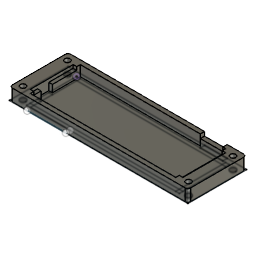
case-bottom (Autodesk Fusion 360 design; units mm, degrees)
part number: 2025-11-21-15-01-15-450
part number: 2025-11-21-15-01-59-170
Autodesk Fusion 360 part; units mm, degrees
sketch "Sketch1" plane through (0, 0, 0) normal (0, 0, 1) x (1, 0, 0) in component "guilty pad case"
  line L0 (0, 0) -> (94.784, 0)
  line L1 (94.784, 0) -> (94.784, -31)
  line L2 (94.784, -31) -> (0, -31)
  line L3 (0, -31) -> (0, 0)
  line L4 (-8, 2.7) -> (102.784, 2.7)
  line L5 (102.784, 2.7) -> (102.784, -33.7)
  line L6 (102.784, -33.7) -> (-8, -33.7)
  line L7 (-8, -33.7) -> (-8, 2.7)
  circle A0 centre (-4, -29.3) radius 1.7
  circle A1 centre (98.784, -29.3) radius 1.7
  circle A2 centre (98.784, -1.7) radius 1.7
  circle A3 centre (-4, -1.7) radius 1.7
  line L8 (3, -31) -> (27, -31)
  line L9 (27, -33.7) -> (3, -33.7)
  line L10 (90.784, 0) -> (76.784, 0)
  line L11 (76.784, 0) -> (76.784, 2.7)
  line L12 (76.784, 2.7) -> (90.784, 2.7)
  line L13 (90.784, 2.7) -> (90.784, 0)
  line L14 (92.534, 0) -> (92.534, -31)
  line L15 (2.25, 0) -> (2.25, -31)
  line L16 (0, -2.2) -> (94.784, -2.2)
  line L17 (0, -28.8) -> (94.784, -28.8)
  line L18 (0, -24.3) -> (2.25, -24.3)
  line L19 (0, -17.3) -> (2.25, -17.3)
  dimension "d4" = 36.4
  dimension "d5" = 110.784
  dimension "d6" = 94.784
  dimension "d7" = 31
  dimension "d9" = 3.4
  dimension "d10" = 4.4
  dimension "d11" = 4
  dimension "d12" = 3.4
  dimension "d13" = 4
  dimension "d14" = 4.4
  dimension "d15" = 3.4
  dimension "d16" = 4.4
  dimension "d17" = 4
  dimension "d18" = 3.4
  dimension "d19" = 4.4
  dimension "d20" = 4
  dimension "d21" = 2.7
  dimension "d22" = 8
  dimension "d23" = 24
  dimension "d24" = 2.7
  dimension "d26" = 4
  dimension "d27" = 14
  dimension "d32" = 2.25
  dimension "d33" = 2.25
  dimension "d73" = 2.2
  dimension "d74" = 2.2
  dimension "d77" = 4.5
  dimension "d78" = 7
  constraint horizontal L0
  constraint vertical L1
  constraint horizontal L2
  constraint vertical L3
  constraint coincident L0.start L3.end
  constraint horizontal L4
  constraint vertical L5
  constraint horizontal L6
  constraint vertical L7
  constraint horizontal L8
  constraint horizontal L9
  constraint coincident L2 L8.start
  constraint horizontal L10
  constraint vertical L11
  constraint horizontal L12
  constraint vertical L13
  constraint coincident L4 L11.end
  constraint coincident L0 L10.start
  constraint coincident L0 L14.start
  constraint coincident L2 L14.end
  constraint perpendicular L2 L14
  constraint coincident L0 L15.start
  constraint coincident L2 L15.end
  constraint perpendicular L2 L15
  constraint coincident L3 L16.start
  constraint coincident L1 L16.end
  constraint perpendicular L1 L16
  constraint coincident L3 L17.start
  constraint coincident L1 L17.end
  constraint perpendicular L1 L17
  constraint coincident L3 L18.start
  constraint coincident L15 L18.end
  constraint perpendicular L15 L18
  constraint coincident L3 L19.start
  constraint coincident L15 L19.end
  constraint perpendicular L15 L19
  measures "d4" distance of L4.start L6.end
  measures "d5" distance of L4.start L4.end
  measures "d6" distance of L0.start L0.end
  measures "d7" distance of L0.start L2.end
  measures "d9" diameter of A0
  measures "d10" distance of L6 A0.centre
  measures "d11" distance of L7 A0.centre
  measures "d12" diameter of A1
  measures "d13" distance of L5 A1.centre
  measures "d14" distance of L6 A1.centre
  measures "d15" diameter of A2
  measures "d16" distance of L4 A2.centre
  measures "d17" distance of L5 A2.centre
  measures "d18" diameter of A3
  measures "d19" distance of L4 A3.centre
  measures "d20" distance of L7 A3.centre
  measures "d21" distance of L2 L6
  measures "d22" distance of L1 L5
  measures "d23" distance of L8.start L8.end
  measures "d24" distance of L8.end L9.start
  measures "d26" distance of L0.end L13
  measures "d27" distance of L11 L13
  measures "d32" distance of L1 L14
  measures "d33" distance of L3 L15
  measures "d73" distance of L0 L16
  measures "d74" distance of L2 L17
  measures "d77" distance of L17 L18
  measures "d78" distance of L18 L19
extrude "Extrude2" add sketch "Sketch1" along normal blind 7.5 contours L0 L1 L2 L3 L4 L5 L6 L7 L8 L9 L11 L13 | L0 L3 L15 L16 | L0 L1 L14 L16 | L1 L2 L14 L17 | L2 L3 L15 L17 makes body 1 in component "guilty pad case"
extrude "Extrude3" add sketch "Sketch1" along normal blind 5.5 separate body contours L0 L3 L15 L16 | L3 L15 L16 L19 | L1 L14 L16 L17 | L0 L1 L14 L16 | L3 L15 L17 L18 | L1 L2 L14 L17 | L2 L3 L15 L17 makes body 2 at (0, -11.5333, 1.8333) makes body 3 at (94.784, -10.3333, 1.8333) makes body 4 at (0, -28.7667, 1.8333) in component "guilty pad case"
extrude "Extrude9" add sketch "Sketch1" along normal blind 1 contours L0 L1 L2 L3 L4 L5 L6 L7 L8 L9 L11 L13 | L0 L3 L15 L16 | L0 L10 L14 L15 L16 | L3 L15 L16 L19 | L0 L4 L10 L11 L12 L13 | L14 L15 L16 L17 | L3 L15 L18 L19 | L1 L14 L16 L17 | L0 L1 L14 L16 | L3 L15 L17 L18 | L1 L2 L14 L17 | L2 L8 L14 L15 L17 | L2 L3 L15 L17 | A0 | A1 | A2 | A3 bodies 2 4 1 3 in component "guilty pad case"
fillet "Fillet2" radius 1.7 4 edges at (-8, -33.7, 3.75) (-8, 2.7, 3.75) (102.784, 2.7, 3.75) (102.784, -33.7, 3.75) on bodies 2 in component "guilty pad case"
extrude "Extrude13" add sketch "Sketch1" along normal blind 5 separate body contours L0 L4 L10 L11 L12 L13 makes body 5 in component "guilty pad case"
component "guilty pad case" placed x (1, 0, 0) y (0, 1, 0) z (0, 0, 1) at (0, 0, 0)
